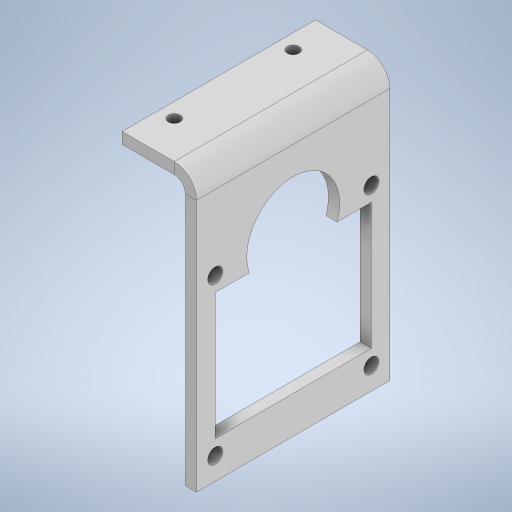
# Autodesk Inventor part: neck_joint
Saved by Autodesk Inventor 2024.1 (Build 281209000, 209)
## iProperties
Created: 2024-10-11
Part Number: neck_joint
Material: 一般
Document SubType Name: Sheet Metal
Designer: hibik
Density: 1 g/cm^3
Sheet Metal Rule: Default_mm
Appearance: 既定
Author: hibik
Autodesk Inventor part; units mm, degrees
ref_plane "YZ Plane" through (0, 0, 0) normal (1, 0, 0) x (0, 1, 0)
ref_plane "XZ Plane" through (0, 0, 0) normal (0, 1, 0) x (-1, 0, 0)
ref_plane "XY Plane" through (0, 0, 0) normal (0, 0, 1) x (1, 0, 0)
sketch "スケッチ1" plane through (0, 0, 0) normal (1, 0, 0) x (0, 1, 0)
  circle A0 centre (0, 0) radius 6.25
  line L0 (0, 13) -> (-24, 13)
  line L1 (-24, 13) -> (-24, -13)
  line L2 (-24, -13) -> (0, -13)
  line L3 (0, -13) -> (0, 13) construction
  line L4 (0, 13) -> (13, 13)
  line L5 (13, 13) -> (13, -13)
  line L6 (13, -13) -> (0, -13)
  line L7 (0, -13) -> (0, 13)
  dimension "d0" = 12.5
  dimension "d1" = 24
  dimension "d2" = 26
  dimension "d3" = 13
  measures "d0" diameter of A0
  measures "d1" distance of L2.end L1.end
  measures "d2" distance of L1.end L0.end
  measures "d3" distance between parallel lines of L3 L5
extrude "プレート1" add sketch "スケッチ1" along normal blind 1.5 contours A0 L7 L4 L5 L6 | A0 L7 L2 L1 L0
sketch "スケッチ2" plane through (1.5, 11.5, -13) normal (0, 1, 0) x (-1, 0, 0)
  line L0 (0, 26) -> (0, 0)
  line L1 (0, 0) -> (10, 0)
  line L2 (10, 0) -> (10, 26)
  line L3 (10, 26) -> (0, 26)
  constraints: 6 end point, 1 horizontal, 1 perpendicular, 1 vertical
edge flange "フランジ1" height 10 angle 90 thickness 1.5 bend radius 1.5 thickness toward (0, 1, 0) relief straight relief width 1.5 relief depth 0.75 edges at (0, 13, 0) wall of the first edge with corners at (1.5, 11.5, 13) (1.5, 11.5, -13) (-8.5, 11.5, -13) (-8.5, 11.5, 13)
bend "曲げ1"
corner "コーナー1"
sketch "スケッチ3" plane through (1.5, 0, 0) normal (1, 0, 0) x (0, 0, -1)
  circle A0 centre (10.5, 0) radius 1 projected
  circle A1 centre (-10.5, 0) radius 1 projected
  circle A2 centre (-10.5, -21) radius 1 projected
  circle A3 centre (10.5, -21) radius 1 projected
  point P0 (0, 0)
extrude "切り取り1" cut sketch "スケッチ3" against normal blind 1.5
sketch "スケッチ4" plane through (1.5, 0, 0) normal (1, 0, 0) x (0, 0, -1)
  circle A0 centre (-10.5, -21) radius 1 projected
  circle A1 centre (10.5, 0) radius 1 projected
  circle A2 centre (-10.5, 0) radius 1 projected
  circle A3 centre (10.5, -21) radius 1 projected
  line L0 (13, 10) -> (-13, 10) projected
  line L1 (-13, -24) -> (-13, 10) projected
  line L2 (13, -24) -> (-13, -24) projected
  line L3 (13, 10) -> (13, -24) projected
  circle A4 centre (0, 0) radius 6.25 projected
  line L4 (-10.5, 0) -> (10.5, 0)
  line L5 (10.5, 0) -> (10.5, -21)
  line L6 (10.5, -21) -> (-10.5, -21)
  line L7 (-10.5, -21) -> (-10.5, 0)
  line L8 (-10.5, -2) -> (10.5, -2)
  line L9 (10.5, -2) -> (10.5, -19)
  line L10 (10.5, -19) -> (-10.5, -19)
  line L11 (-10.5, -19) -> (-10.5, -2)
  dimension "d17" = 2
  dimension "d18" = 2
  constraints: 16 end point, 4 parallel, 2 horizontal, 2 perpendicular, 2 point on line
  measures "d17" distance between parallel lines of L4 L8
  measures "d18" distance between parallel lines of L6 L10
extrude "切り取り2" cut sketch "スケッチ4" against normal blind 1.5 contours L7 L8 A4 L5 L10 | L8 A4
sketch "スケッチ5" plane through (-8.5, 13, 13) normal (0, 1, 0) x (1, 0, 0)
  circle A0 centre (2, 21) radius 0.8
  circle A1 centre (2, 5) radius 0.8
  line L0 (0, 0) -> (0, 26) projected
  line L1 (0, 26) -> (7, 26) projected
  line L2 (7, 0) -> (0, 0) projected
  point P0 (8.5, 13)
  dimension "d21" = 1.6
  dimension "d23" = 2
  dimension "d24" = 5
  dimension "d25" = 5
  constraints: 2 centre point, 1 equal radius, 1 vertical alignment
  measures "d21" diameter of A0
  measures "d23" distance from line of L0 A0.centre
  measures "d24" distance from line of L1 A0.centre
  measures "d25" distance from line of L2 A1.centre
extrude "切り取り3" cut sketch "スケッチ5" against normal blind 1.5
equation "\"d15\" = Thickness"
equation "\"d18\" = d17"
equation "\"d19\" = Thickness"
equation "\"d25\" = d24"
equation "\"d26\" = Thickness"
equation "\"d4\" = Thickness"
equation "\"d5\" = BendReliefWidth"
equation "\"d6\" = BendReliefDepth"
equation "\"d7\" = MinimumRemnant"
equation "\"d8\" = TransitionRadius"
equation "\"d11\" = BendRadius"
equation "\"d12\" = CornerReliefSize"
equation "\"d13\" = GapSize"
equation "\"d14\" = JacobiRadiusSize"
equation "\"BendRadius\" = Thickness"
equation "\"BendReliefWidth\" = Thickness"
equation "\"BendReliefDepth\" = 0.5 * Thickness"
equation "\"CornerReliefSize\" = 4 * Thickness"
equation "\"MinimumRemnant\" = 2 * Thickness"
equation "\"TransitionRadius\" = BendRadius"
equation "\"JacobiRadiusSize\" = BendRadius"
equation "\"GapSize\" = Thickness"
equation "\"Thickness\" = 1.5"
